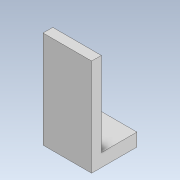
# Autodesk Inventor part: battery_fix_board
Saved by Autodesk Inventor 2020 (Build 240168000, 168)
## iProperties
Created: 2021-01-16
Part Number: battery_fix_board
Material: Generic
Document SubType Name: Modeling
Designer: DELL
Density: 1 g/cm^3
Appearance: Default
Author: DELL
Autodesk Inventor part; units mm, degrees
ref_plane "YZ Plane" through (0, 0, 0) normal (1, 0, 0) x (0, 1, 0)
ref_plane "XZ Plane" through (0, 0, 0) normal (0, 1, 0) x (-1, 0, 0)
ref_plane "XY Plane" through (0, 0, 0) normal (0, 0, 1) x (1, 0, 0)
sketch "Sketch1" plane through (0, 0, 0) normal (1, 0, 0) x (0, 1, 0)
  line L0 (30, 0) -> (0, 0)
  line L1 (0, 0) -> (0, -14)
  line L2 (0, -14) -> (4, -14)
  line L3 (4, -14) -> (4, -3)
  line L4 (4, -3) -> (30, -3)
  line L5 (30, -3) -> (30, 0)
  dimension "d0" = 4
  dimension "d1" = 14
  dimension "d2" = 3
  dimension "d3" = 30
  constraints: 12 end point, 5 perpendicular, 1 horizontal
  measures "d0" distance between parallel lines of L1 L3
  measures "d1" distance between parallel lines of L0 L2
  measures "d2" distance between parallel lines of L0 L4
  measures "d3" distance between parallel lines of L1 L5
extrude "Extrusion1" add sketch "Sketch1" against normal mid plane 15
sketch "Sketch2" plane through (-7.5, 4, -14) normal (0, 1, 0) x (1, 0, 0)
  circle A0 centre (7.5, -7.5) radius 1.25
  line L0 (0, 0) -> (15, 0) projected
  line L1 (0, -14) -> (15, -14) projected
  line L2 (0, -11) -> (15, -11) projected
  point P0 (7.5, -14)
  point P1 (7.5, -14)
  dimension "d6" = 2.5
  dimension "d10" = 3.5
  constraints: 1 centre point, 1 midpoint, 1 vertical alignment
  measures "d6" diameter of A0
  measures "d10" distance from line of L2 A0.centre
extrude "Extrusion2" cut sketch "Sketch2" against normal through all
body "Solid1"
